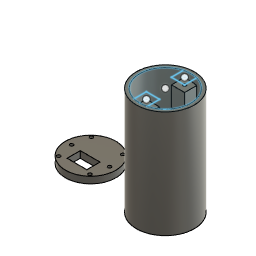
SM_Casing v12 (Autodesk Fusion 360 design; units mm, degrees)
Autodesk Fusion 360 part; units mm, degrees
sketch "base" plane through (0, 0, 0) normal (0, 1, 0) x (1, 0, 0)
  circle A0 centre (19.2659, 18.0126) radius 17.5
  circle A1 centre (19.2659, 18.0126) radius 15.5
  circle A2 centre (9.7659, 27.9536) radius 1
  circle A3 centre (9.7659, 8.0716) radius 1
  circle A4 centre (28.7659, 8.0716) radius 1
  circle A5 centre (28.2659, 28.4536) radius 1
  line L0 (32.2659, 9.5716) -> (26.7659, 9.5716)
  line L1 (11.7659, 9.5716) -> (6.2659, 9.5716)
  line L2 (26.7659, 31.5773) -> (26.7659, 26.4536)
  line L3 (26.7659, 9.5716) -> (26.7659, 4.4479)
  line L4 (11.7659, 31.5773) -> (11.7659, 26.4536)
  line L5 (11.7659, 9.5716) -> (11.7659, 4.4479)
  line L6 (6.2659, 26.4536) -> (11.7659, 26.4536)
  line L7 (26.7659, 26.4536) -> (32.2659, 26.4536)
  line L8 (26.9331, 22.0126) -> (26.9331, 14.0126)
  line L9 (11.7659, 22.0126) -> (11.7659, 14.0126)
  line L10 (4.2909, 22.0126) -> (11.7659, 22.0126)
  line L11 (26.9331, 22.0126) -> (34.2408, 22.0126)
  line L12 (4.2909, 14.0126) -> (11.7659, 14.0126)
  line L13 (26.9331, 14.0126) -> (34.2408, 14.0126)
  circle A6 centre (7.7659, 18) radius 1
  circle A7 centre (30.9331, 17.9842) radius 1
  line L14 (6.7891, 10.2061) -> (31.7891, 10.2061)
  line L15 (31.7891, 10.2061) -> (31.7891, 12.2061)
  line L16 (31.7891, 12.2061) -> (6.7891, 12.2061)
  line L17 (6.7891, 12.2061) -> (6.7891, 10.2061)
  dimension "d18" = 2
  dimension "d21" = 2
  dimension "d37" = 31
  dimension "d38" = 35
  dimension "d39" = 2
  dimension "d40" = 1.5
  dimension "d43" = 2
  dimension "d45" = 4
  dimension "d48" = 25
  dimension "d49" = 2
  constraint concentric A0 A1
  constraint coincident A1 L4.start
  constraint coincident A1 L5.end
  constraint coincident A1 L2.start
  constraint coincident A1 L3.end
  constraint coincident A1 L6.start
  constraint coincident A1 L7.end
  constraint perpendicular L4 L6
  constraint coincident A1 L0.start
  constraint coincident A1 L1.end
  constraint coincident L0.end L2
  constraint coincident L1.start L4
  constraint collinear L0 L1
  constraint coincident L2.end L6
  constraint collinear L2 L3
  constraint collinear L4 L5
  constraint collinear L6 L7
  constraint coincident A1 L10.start
  constraint coincident A1 L11.end
  constraint parallel L6 L10
  constraint coincident A1 L12.start
  constraint coincident A1 L13.end
  constraint horizontal L12
  constraint coincident L8.start L10
  constraint coincident L8.end L12
  constraint perpendicular L8 L12
  constraint perpendicular L9 L12
  constraint collinear L10 L11
  constraint collinear L12 L13
  constraint horizontal L14
  constraint vertical L15
  constraint horizontal L16
  constraint vertical L17
  measures "d18" diameter of A2
  measures "d21" diameter of A5
  measures "d37" diameter of A1
  measures "d38" diameter of A0
  measures "d39" distance of A2.centre L4
  measures "d40" distance of A2.centre L6
  measures "d43" diameter of A6
  measures "d45" distance of L9 A6.centre
  measures "d48" distance of L14.start L14.end
  measures "d49" distance of L14.end L15.end
extrude "Extrude1" add sketch "base" along normal blind 35 contours A0 makes body 1
extrude "Extrude2" add sketch "base" along normal blind 4 contours A1 L0 L1 L2 L3 L4 L5 L6 L7 L8 L9 L10 L11 L12 L13 bodies 1
extrude "Extrude3" add sketch "base" along normal blind 30 contours A1 L8 L11 L13 | A1 L2 L7 | A1 L0 L3 | A1 L4 L6 | A1 L1 L5 | A1 L9 L10 L12 | A2 | A3 | A4 | A5 | A6 | A7 bodies 1
extrude "Extrude4" add sketch "base" along normal blind 35 separate body contours A6 | A7 makes body 2 at (7.1042, 23.3333, -17.2502) makes body 3 at (31.9281, 23.3333, -17.8846)
extrude "Extrude5" cut 1 faces at (30.3443, 35, -17.8612) along direction (0, -1, 0) blind 10 on bodies 3 bodies 1 3
extrude "Extrude6" cut 1 faces at (8.0699, 35, -17.8057) along direction (0, -1, 0) blind 10 on bodies 2 bodies 1 2
extrude "Extrude7" add sketch "base" along normal blind 35 separate body contours A2 makes body 4
extrude "Extrude8" cut 1 faces at (10.0231, 35, -27.8122) along direction (0, -1, 0) blind 10 on bodies 4 bodies 1 4
extrude "Extrude9" add sketch "base" along normal blind 35 separate body contours A3 | A4 | A5 makes body 5 at (29.7609, 23.3333, -7.9721) makes body 6 at (10.7609, 23.3333, -7.9721) makes body 7 at (29.2609, 23.3333, -28.354)
extrude "Extrude10" cut 3 faces at (28.5948, 35, -8.3894) (27.6322, 35, -28.5982) (10.0413, 35, -8.16) along direction (0, -1, 0) blind 10 on bodies 5 6 7 bodies 1 5 6 7
combine "Combine1" operation add target body 1 tool bodies 2 3 4 5 6 7
sketch "base-cap" plane through (0, 0, 0) normal (0, 1, 0) x (1, 0, 0)
  circle A0 centre (-29, 21) radius 15.25
  circle A1 centre (-19.5001, 11.0587) radius 1
  circle A2 centre (-38.4996, 11.0589) radius 1
  circle A3 centre (-19.9992, 31.4408) radius 1
  circle A4 centre (-38.4993, 30.9417) radius 1
  line L0 (-22.8216, 12.5024) -> (-34.8216, 12.5024)
  line L1 (-34.8216, 12.5024) -> (-34.8216, 20.5024)
  line L2 (-34.8216, 20.5024) -> (-22.8216, 20.5024)
  line L3 (-22.8216, 20.5024) -> (-22.8216, 12.5024)
  circle A5 centre (-40.5, 20.9864) radius 1
  circle A6 centre (-17.5, 21.008) radius 1
  dimension "d77" = 30.5
  dimension "d78" = 2
  dimension "d79" = 2
  dimension "d80" = 2
  dimension "d81" = 2
  dimension "d84" = 12
  dimension "d85" = 8
  dimension "d92" = 2
  dimension "d93" = 2
  constraint horizontal L0
  constraint vertical L1
  constraint horizontal L2
  constraint vertical L3
  measures "d77" diameter of A0
  measures "d78" diameter of A1
  measures "d79" diameter of A2
  measures "d80" diameter of A3
  measures "d81" diameter of A4
  measures "d84" distance of L0.start L0.end
  measures "d85" distance of L0.end L1.end
  measures "d92" diameter of A5
  measures "d93" diameter of A6
extrude "Extrude11" add sketch "base-cap" along normal blind 4 separate body contours A0 | L0 L1 L2 L3 | A5 | A6 makes body 8
extrude "Extrude14" cut sketch "base-cap" along normal blind 4 contours L0 L1 L2 L3 bodies 8
extrude "Extrude15" cut sketch "base-cap" along normal blind 4 contours A6 bodies 8
extrude "Extrude16" cut sketch "base-cap" along normal blind 4 contours A5 bodies 8
extrude "Extrude17" add 1 faces at (35.9763, 35, -16.3731) along direction (0, 1, 0) blind 30 on bodies 1 bodies 1
sketch "Sketch6" plane through (0, 65, 0) normal (0, 1, 0) x (-1, 0, 0)
  circle A0 centre (-19.2659, -18.0126) radius 15.5
  circle A1 centre (-19.2659, -18.0126) radius 17.5
  circle A2 centre (-19.2659, -18.0126) radius 15.5
  line L0 (-23.2651, -32.9878) -> (-23.2651, -25.6867)
  line L1 (-23.2651, -25.6867) -> (-15.2651, -25.6867)
  line L2 (-15.2651, -25.6867) -> (-15.2651, -32.9874)
  line L3 (-23.2785, -3.041) -> (-23.2785, -10.5081)
  line L4 (-23.2785, -10.5081) -> (-15.2785, -10.5081)
  line L5 (-15.2785, -10.5081) -> (-15.2785, -3.0343)
  circle A3 centre (-19.2804, -6.5081) radius 1
  circle A4 centre (-19.2992, -29.6867) radius 1
  dimension "d102" = 31
  dimension "d103" = 2
  dimension "d104" = 2
  dimension "d105" = 8
  dimension "d106" = 8
  dimension "d107" = 4
  dimension "d108" = 4
  constraint coincident A2 L0.start
  constraint perpendicular L0 L1
  constraint coincident A2 L2.end
  constraint perpendicular L1 L2
  constraint coincident A2 L3.start
  constraint parallel L2 L3
  constraint perpendicular L2 L4
  constraint coincident A2 L5.end
  constraint perpendicular L4 L5
  measures "d102" diameter of A2
  measures "d103" diameter of A3
  measures "d104" diameter of A4
  measures "d105" distance of L0.end L1.end
  measures "d106" distance of L3.end L4.end
  measures "d107" distance of L4 A3.centre
  measures "d108" distance of L1 A4.centre
extrude "Extrude18" add sketch "Sketch6" against normal blind 16 contours A0 A2 L3 L4 L5 | A0 A2 L0 L1 L2 | A3 | A4 bodies 1
extrude "Extrude19" cut sketch "Sketch6" against normal blind 4 contours A0 A2 L3 L4 L5 | A0 A2 L0 L1 L2 | A3 | A4 bodies 1
extrude "Extrude20" cut sketch "Sketch6" against normal blind 11 contours A3 | A4 bodies 1
sketch "Sketch3" plane through (0, 0, 0) normal (0, 1, 0) x (1, 0, 0)
  circle A0 centre (58.9844, 20.3053) radius 15.6723
  circle A1 centre (49.5237, 30.2998) radius 1
  circle A2 centre (68.0213, 30.7869) radius 1
  circle A3 centre (47.4889, 20.3054) radius 1
  circle A4 centre (70.7523, 20.3426) radius 1
  circle A5 centre (49.5127, 10.4099) radius 1
  circle A6 centre (68.5221, 10.411) radius 1
  dimension "d71" = 2
  dimension "d72" = 2
  dimension "d73" = 2
  dimension "d74" = 2
  dimension "d75" = 2
  dimension "d76" = 2
  measures "d71" diameter of A1
  measures "d72" diameter of A2
  measures "d73" diameter of A3
  measures "d74" diameter of A4
  measures "d75" diameter of A5
  measures "d76" diameter of A6
named bodies: "base", "base-cap"
